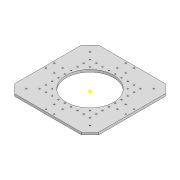
# Autodesk Inventor part: RobotBase
Saved by Autodesk Inventor 2022 (Build 260153000, 153)
## iProperties
Created: 2022-10-20
Part Number: RobotBase
Material: Generic
Document SubType Name: Modeling
Designer: MVeszpremi
Density: 1 g/cm^3
Appearance: Default
Author: MVeszpremi
Autodesk Inventor part; units mm, degrees
ref_plane "YZ Plane" through (0, 0, 0) normal (1, 0, 0) x (0, 1, 0)
ref_plane "XZ Plane" through (0, 0, 0) normal (0, 1, 0) x (-1, 0, 0)
ref_plane "XY Plane" through (0, 0, 0) normal (0, 0, 1) x (1, 0, 0)
sketch "Sketch1" plane through (0, 0, 0) normal (0, 1, 0) x (-1, 0, 0)
  point P0 (0, 0)
sketch "Sketch2" plane through (0, 0, 0) normal (0, 1, 0) x (-1, 0, 0)
  line L0 (-100, 100) -> (100, 100)
  line L1 (100, 100) -> (100, -100)
  line L2 (100, -100) -> (-100, -100)
  line L3 (-100, -100) -> (-100, 100)
  line L4 (-100, 100) -> (100, -100) construction
  line L5 (100, 100) -> (-100, -100) construction
  line L6 (95, 10) -> (75, 10)
  line L7 (75, 10) -> (75, -10)
  line L8 (75, -10) -> (95, -10)
  line L9 (95, -10) -> (95, 10)
  line L10 (95, 10) -> (75, -10) construction
  line L11 (75, 10) -> (95, -10) construction
  circle A0 centre (95, 10) radius 1.5
  circle A1 centre (95, -10) radius 1.5
  circle A2 centre (75, -10) radius 1.5
  circle A3 centre (75, 10) radius 1.5
  line L12 (-10, 95) -> (-10, 75)
  circle A4 centre (-10, 95) radius 1.5
  circle A5 centre (-10, 75) radius 1.5
  line L13 (-10, 75) -> (10, 75)
  line L14 (10, 75) -> (10, 95)
  line L15 (-10, 75) -> (10, 95) construction
  line L16 (-10, 95) -> (10, 75) construction
  line L17 (10, 95) -> (-10, 95)
  circle A6 centre (10, 95) radius 1.5
  circle A7 centre (10, 75) radius 1.5
  line L18 (-95, -10) -> (-75, -10)
  circle A8 centre (-95, -10) radius 1.5
  circle A9 centre (-75, -10) radius 1.5
  line L19 (-75, -10) -> (-75, 10)
  line L20 (-75, 10) -> (-95, 10)
  line L21 (-75, -10) -> (-95, 10) construction
  line L22 (-95, -10) -> (-75, 10) construction
  line L23 (-95, 10) -> (-95, -10)
  circle A10 centre (-95, 10) radius 1.5
  circle A11 centre (-75, 10) radius 1.5
  line L24 (10, -95) -> (10, -75)
  circle A12 centre (10, -95) radius 1.5
  circle A13 centre (10, -75) radius 1.5
  line L25 (10, -75) -> (-10, -75)
  line L26 (-10, -75) -> (-10, -95)
  line L27 (10, -75) -> (-10, -95) construction
  line L28 (10, -95) -> (-10, -75) construction
  line L29 (-10, -95) -> (10, -95)
  circle A14 centre (-10, -95) radius 1.5
  circle A15 centre (-10, -75) radius 1.5
  point P0 (0, 0)
  point P1 (85, 0)
  point P2 (0, 85)
  point P3 (-85, 0)
  point P4 (0, -85)
  dimension "d0" = 200
  dimension "d1" = 200
  dimension "d2" = 20
  dimension "d3" = 20
  dimension "d4" = 5
  dimension "d5" = 3
  dimension "d6" = 3
  dimension "d7" = 3
  dimension "d8" = 3
  dimension "d11" = 360
  constraints: 60 end point, 16 centre point, 16 coincident, 10 midpoint, 4 parallel, 2 horizontal, 2 perpendicular, 77 other
  measures "d0" distance of L0.end L1.end
  measures "d1" distance of L1.end L2.end
  measures "d2" distance of L8.end L6.start
  measures "d3" distance of L7.end L8.end
  measures "d4" distance between parallel lines of L1 L9
  measures "d5" diameter of A0
  measures "d6" diameter of A1
  measures "d7" diameter of A2
  measures "d8" diameter of A3
extrude "Extrusion1" add sketch "Sketch2" along normal blind 5.4 contours L0 L1 L2 L3 | L6 A0 L9 A1 L8 A2 L7 A3 | A4 L17 A6 L14 A7 L13 A5 L12 | A8 L23 A10 L20 A11 L19 A9 L18 | A12 L29 A14 L26 A15 L25 A13 L24
chamfer "Chamfer1" distance 20 angle 45 4 edges at (100, 2.7, -100) (-100, 2.7, -100) (100, 2.7, 100) (-100, 2.7, 100)
sketch "Sketch5" plane through (0, 0, 0) normal (0, -1, 0) x (1, 0, 0)
  circle A0 centre (0, 0) radius 4
  circle A1 centre (0, 0) radius 1.45
  dimension "d32" = 2.9
  dimension "d33" = 8
  constraints: 2 centre point, 2 coincident
  measures "d32" diameter of A1
  measures "d33" diameter of A0
extrude "Extrusion3" cut sketch "Sketch5" against normal blind 8 contours A1
pattern_linear "Rectangular Pattern1" count 5 spacing 15 along (1, 0, 0) count 5 spacing 15 along (0, 0, 1) of "Extrusion3"
mirror "Mirror1" about plane through (0, 0, 0) normal (1, 0, 0) of "Extrusion3", "Rectangular Pattern1"
mirror "Mirror2" about plane through (0, 0, 0) normal (0, 0, 1) of "Extrusion3", "Rectangular Pattern1", "Mirror1"
sketch "Sketch6" plane through (0, 5.4, 0) normal (0, 1, 0) x (1, 0, 0)
  line L0 (-100, 80) -> (-80, 100) projected
  line L1 (-90, 90) -> (-75.8579, 75.8579)
  circle A0 centre (-75.8579, 75.8579) radius 1.5
  point P0 (0, 0)
  dimension "d44" = 3
  dimension "d45" = 20
  constraints: 2 end point, 1 centre point, 1 coincident, 1 midpoint, 1 perpendicular
  measures "d44" diameter of A0
  measures "d45" distance of L1.start L1.end
extrude "Extrusion5" cut sketch "Sketch6" against normal blind 16
pattern_circular "Circular Pattern1" count 4 over 360 about axis through (0, 0, 0) along (0, 1, 0) of "Extrusion5"
sketch "Sketch7" plane through (0, 5.4, 0) normal (0, 1, 0) x (1, 0, 0)
  circle A0 centre (0, 0) radius 1.45 projected
  circle A1 centre (0, 0) radius 56
  dimension "d51" = 112
  constraints: 1 centre point, 1 coincident
  measures "d51" diameter of A1
extrude "Extrusion6" cut sketch "Sketch7" against normal blind 10
equation "\"d34\" = d33"
body "Solid1"
